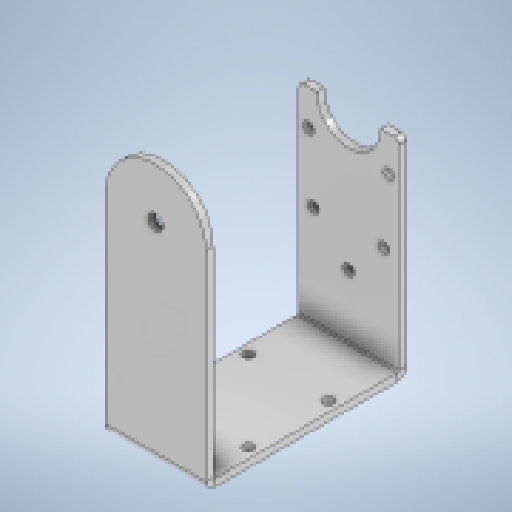
# Autodesk Inventor part: axis_9_bottom_frame
Saved by Autodesk Inventor 2025.2 (Build 292293000, 293)
## iProperties
Created: 2025-05-04
Part Number: axis_9_bottom_frame
Material: Aluminum 6061-AHC
Document SubType Name: Sheet Metal
Designer: User
Density: 2.7 g/cm^3
Sheet Metal Rule: Default_mm
Appearance: Aluminum - Dark
Author: User
Autodesk Inventor part; units mm, degrees
ref_plane "YZ Plane" through (0, 0, 0) normal (1, 0, 0) x (0, 1, 0)
ref_plane "XZ Plane" through (0, 0, 0) normal (0, 1, 0) x (-1, 0, 0)
ref_plane "XY Plane" through (0, 0, 0) normal (0, 0, 1) x (1, 0, 0)
sketch "Sketch1" plane through (0, 0, 0) normal (0, 1, 0) x (-1, 0, 0)
  line L0 (10, -18.5) -> (-10, -18.5)
  line L1 (-10, -18.5) -> (-10, 18.5)
  line L2 (-10, 18.5) -> (10, 18.5)
  line L3 (10, 18.5) -> (10, -18.5)
  point P0 (0, 0)
  dimension "d0" = 20
  dimension "d1" = 37
  dimension "d2" = 18.5
  dimension "d3" = 10
  measures "d0" distance of L0.start L0.end
  measures "d1" distance of L0.end L1.end
  measures "d2" distance from line of L0 point (0, 0)
  measures "d3" distance from line of point (0, 0) L3
extrude "Plate1" add sketch "Sketch1" along normal blind 1.5
sketch "Sketch2" plane through (-10, 0, -20) normal (0, 0, 1) x (1, 0, 0)
  line L0 (20, 0) -> (0, 0)
  line L1 (0, 0) -> (0, 51.6)
  line L2 (0, 51.6) -> (20, 51.6)
  line L3 (20, 51.6) -> (20, 0)
  constraints: 8 end point
edge flange "Flange1" height 51.6 angle 90 thickness 1.5 bend radius 0.31 thickness toward (0, 0, 1) relief straight relief width 1.5 relief depth 0.75 edges at (0, 1.5, -18.5) wall of the first edge with corners at (10, 0, -20) (-10, 0, -20) (-10, 51.6, -20) (10, 51.6, -20)
bend "Bend1"
corner "Corner1"
sketch "Sketch3" plane through (10, 0, 20) normal (0, 0, -1) x (-1, 0, 0)
  line L0 (20, 0) -> (0, 0)
  line L1 (0, 0) -> (0, 51.6)
  line L2 (0, 51.6) -> (20, 51.6)
  line L3 (20, 51.6) -> (20, 0)
  constraints: 8 end point
edge flange "Flange2" height 51.6 angle 90 thickness 1.5 bend radius 0.31 thickness toward (0, 0, -1) relief straight relief width 1.5 relief depth 0.75 edges at (0, 1.5, 18.5) wall of the first edge with corners at (-10, 0, 20) (10, 0, 20) (10, 51.6, 20) (-10, 51.6, 20)
bend "Bend2"
corner "Corner2"
sketch "Sketch4" plane through (-10, 51.6, 20) normal (0, 0, 1) x (1, 0, 0)
  circle A0 centre (10, -10) radius 10
  line L0 (0, 0) -> (20, 0) projected
  line L1 (0, 0) -> (20, 0)
  line L2 (20, 0) -> (20, -10)
  line L3 (20, -10) -> (0, -10)
  line L4 (0, -10) -> (0, 0)
  line L5 (0, -49.79) -> (0, 0) projected
  point P0 (10, -51.6)
  point P1 (10, -10)
  point P2 (10, 0)
  point P3 (0, -10)
  point P4 (8.5893, 0)
  point P5 (0, -10)
  dimension "d26" = 20
  dimension "d25" = 10
  dimension "d27" = 10
  dimension "d28" = 10
  constraints: 8 end point, 2 parallel, 1 horizontal, 1 midpoint, 1 perpendicular, 3 other
  measures "d25" distance from line of L0 point (10, -10)
  measures "d27" distance from line of point (10, -10) L2
  measures "d28" distance from line of L5 point (10, -10)
extrude "Extrusion1" cut sketch "Sketch4" against normal blind 10 contours L4 L0 A0 | A0 L0 L2
sketch "Sketch5" plane through (10, 51.6, -20) normal (0, 0, -1) x (-1, 0, 0)
  arc A0 (20, -10) -> (0, -10) centre (10, -10) ccw projected
  point P0 (10, -51.6)
hole "Hole1" at (0, 41.6, -20) direction (0, 0, 1) diameter 12.8 depth 1.5
sketch "Sketch6" plane through (10, 51.6, -20) normal (0, 0, -1) x (-1, 0, 0)
  circle A0 centre (10, -10) radius 6.4 projected
  line L0 (0, 0) -> (20, 0) projected
  line L1 (0, -49.79) -> (0, 0) projected
  line L2 (24, 0) -> (-4, 0)
  line L3 (-4, 0) -> (-4, -9.9)
  line L4 (-4, -9.9) -> (24, -9.9)
  line L5 (24, -9.9) -> (24, 0)
  point P0 (10, -51.6)
  dimension "d38" = 9.9
  dimension "d39" = 4
  dimension "d40" = 28
  constraints: 8 end point, 2 parallel, 1 horizontal, 1 perpendicular, 1 point on line
  measures "d38" distance of L2.end L3.end
  measures "d39" distance between parallel lines of L1 L3
  measures "d40" distance between parallel lines of L5 L3
extrude "Extrusion2" cut sketch "Sketch6" against normal blind 10 contours L4 A0 | A0 L4 L1 L0 L2 L5 | L4 L3 L2 L1 picked at (9.1972, -6.4205)
fillet "Fillet1" radius 1 2 edges at (10, 41.7, -19.25) (-10, 41.7, -19.25)
sketch "Sketch7" plane through (-10, 1.81, 20) normal (0, 0, 1) x (1, 0, 0)
  arc A0 (20, 39.79) -> (0, 39.79) centre (10, 39.79) ccw projected
  point P0 (10, -1.81)
hole "Hole2" at (0, 41.6, 20) direction (0, 0, -1) diameter 3 depth 1.5
sketch "Sketch8" plane through (0, 0, 0) normal (0, -1, 0) x (1, 0, 0)
  line L0 (1.5, 18.5) -> (-1.5, 18.5) projected
  line L1 (-10, 18.5) -> (10, 18.5) projected
  line L2 (10, 18.5) -> (-10, 18.5) projected
  line L3 (10, 18.19) -> (-10, 18.19) projected
  line L4 (-10, -18.19) -> (-10, 18.19) projected
  line L5 (-10, -18.19) -> (10, -18.19) projected
  line L6 (10, 18.19) -> (10, -18.19) projected
  point P0 (0, 0)
  point P1 (8, 9.5)
  point P2 (8, -6.5)
  point P3 (-8, 9.5)
  point P4 (-8, -6.5)
  dimension "d51" = 9
  dimension "d52" = 2
  dimension "d55" = 16
  dimension "d58" = 16
  constraints: 1 horizontal, 1 vertical, 3 other
  measures "d51" distance from line of L1 point (8, 9.5)
  measures "d52" distance from line of L6 point (8, 9.5)
  measures "d55" distance of point (8, 9.5) point (8, -6.5)
  measures "d58" distance of point (8, 9.5) point (-8, 9.5)
hole "Hole3" at (8, 0, 9.5) at (8, 0, -6.5) at (-8, 0, 9.5) at (-8, 0, -6.5) direction (0, 1, 0) diameter 2.1 depth 1.5
sketch "Sketch9" plane through (-10, 1.81, -18.5) normal (0, 0, 1) x (1, 0, 0)
  circle A0 centre (18, 32.89) radius 0.7835 projected
  circle A1 centre (17, 19.67) radius 0.7835 projected
  circle A2 centre (10, 12.37) radius 0.7835 projected
  circle A3 centre (3, 19.67) radius 0.7835 projected
  circle A4 centre (2, 32.89) radius 0.7835 projected
  point P0 (10, -1.81)
hole "Hole4" at (-8, 34.7, -18.5) at (8, 34.7, -18.5) at (7, 21.48, -18.5) at (0, 14.18, -18.5) at (-7, 21.48, -18.5) direction (0, 0, -1) diameter 2.1 depth 1.5
equation "\"d36\" = Thickness"
equation "\"d49\" = Thickness"
equation "\"d66\" = Thickness"
equation "\"d73\" = Thickness"
equation "\"d4\" = Thickness"
equation "\"d5\" = BendReliefWidth"
equation "\"d6\" = BendReliefDepth"
equation "\"d7\" = MinimumRemnant"
equation "\"d8\" = TransitionRadius"
equation "\"d11\" = BendRadius"
equation "\"d12\" = CornerReliefSize"
equation "\"d13\" = GapSize"
equation "\"d14\" = JacobiRadiusSize"
equation "\"d15\" = BendReliefWidth"
equation "\"d16\" = BendReliefDepth"
equation "\"d17\" = MinimumRemnant"
equation "\"d18\" = TransitionRadius"
equation "\"d21\" = BendRadius"
equation "\"d22\" = CornerReliefSize"
equation "\"d23\" = GapSize"
equation "\"d24\" = JacobiRadiusSize"
equation "\"BendReliefWidth\" = Thickness"
equation "\"BendReliefDepth\" = 0.5 * Thickness"
equation "\"CornerReliefSize\" = 4 * Thickness"
equation "\"MinimumRemnant\" = 2 * Thickness"
equation "\"TransitionRadius\" = BendRadius"
equation "\"JacobiRadiusSize\" = BendRadius"
equation "\"GapSize\" = Thickness"
equation "\"Thickness\" = 1.5"
equation "\"BendRadius\" = 0.31"
body "Solid1"
